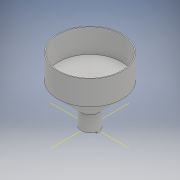
# Autodesk Inventor part: Funnel
Saved by Autodesk Inventor 2017 (Build 210142000, 142)
## iProperties
Created: 2016-05-10
Part Number: Funnel
Material: Generic
Document SubType Name: Modeling
Designer: Bastli
Density: 1 g/cm^3
Appearance: Default
Author: Bastli
Autodesk Inventor part; units mm, degrees
ref_plane "YZ Plane" through (0, 0, 0) normal (1, 0, 0) x (0, 1, 0)
ref_plane "XZ Plane" through (0, 0, 0) normal (0, 1, 0) x (-1, 0, 0)
ref_plane "XY Plane" through (0, 0, 0) normal (0, 0, 1) x (1, 0, 0)
sketch "Sketch1" plane through (0, 0, 0) normal (1, 0, 0) x (0, 1, 0)
  line L0 (10, 0) -> (10, 20)
  line L1 (10, 20) -> (39.5, 49.5)
  line L2 (39.5, 49.5) -> (39.5, 79.5)
  line L3 (0, 79.5) -> (0, 0) construction
  line L4 (10, 20) -> (10, 79.5) construction
  line L5 (39.5, 79.5) -> (40.5, 79.5)
  line L6 (40.5, 79.5) -> (40.5, 49.0858)
  line L7 (40.5, 49.0858) -> (11, 19.5858)
  line L8 (11, 19.5858) -> (11, 0)
  line L9 (11, 0) -> (10, 0)
  dimension "Outlet_Height" = 20
  dimension "Funnel_Angle" = 45
  dimension "Inlet_Diameter" = 79
  dimension "Outlet_Diameter" = 20
  dimension "d23" = 1
  dimension "d24" = 1
  dimension "d25" = 1
  dimension "Inlet_Height" = 30
  constraints: 20 end point, 4 parallel, 2 horizontal, 1 perpendicular, 1 point on line, 1 vertical
  measures "Outlet_Height" distance of L0.start L0.end
  measures "Funnel_Angle" angle of L4 L1
  measures "Inlet_Diameter" diameter of L2 L3
  measures "Outlet_Diameter" diameter of L0 L3
  measures "d23" distance of L2.end L5.end
  measures "d24" distance between parallel lines of L1 L7
  measures "d25" distance between parallel lines of L8 L0
  measures "Inlet_Height" distance of L1.end L2.end
revolve "Revolution1" add sketch "Sketch1" angle 360 about axis through (0, 0, 79.5) along (0, 0, -1)
sketch "Sketch4" plane through (0, 0, 0) normal (0, 0, -1) x (-1, 0, 0)
  line L0 (0, 0) -> (-10.7121, 2.5) construction
  line L1 (0, 0) -> (-48.7838, 0) construction
  line L2 (0, 0) -> (-10.7121, -2.5) construction
  arc A0 (-10.7121, 2.5) -> (-10.7121, -2.5) centre (0, 0) ccw
  line L3 (0, 0) -> (0, 13.9156) construction
  arc A1 (10.7121, -2.5) -> (10.7121, 2.5) centre (0, 0) ccw
  line L4 (-10.7121, 2.5) -> (10.7121, 2.5)
  line L5 (10.7121, -2.5) -> (-10.7121, -2.5)
  circle A2 centre (0, 0) radius 11 projected
  dimension "Bridge_Width" = 5
  constraints: 12 end point, 4 point on circle, 2 centre point, 2 horizontal, 2 symmetric about line, 1 coincident, 1 equal length, 1 parallel, 1 vertical, 4 other
  measures "Bridge_Width" distance between parallel lines of L5 L4
extrude "Extrusion1" add sketch "Sketch4" along normal blind 2 contours L4 A1 L5 A0
sketch "Sketch5" plane through (0, 0, -2) normal (0, 0, -1) x (-1, 0, 0)
  circle A0 centre (0, 0) radius 1.5
  dimension "Bridge_Hole" = 3
  constraints: 1 centre point, 1 coincident
  measures "Bridge_Hole" diameter of A0
extrude "Extrusion2" [suppressed]
fillet "Fillet1" radius 0.5 4 edges at (11, 0, -2) (-11, 0, -2) (0, -2.5, -2) (0, 2.5, -2)
equation "\"d23\" = Wall_Thickness"
equation "\"d24\" = Wall_Thickness"
equation "\"d25\" = Wall_Thickness"
equation "\"Wall_Thickness\" = 1"
body "Solid1"
